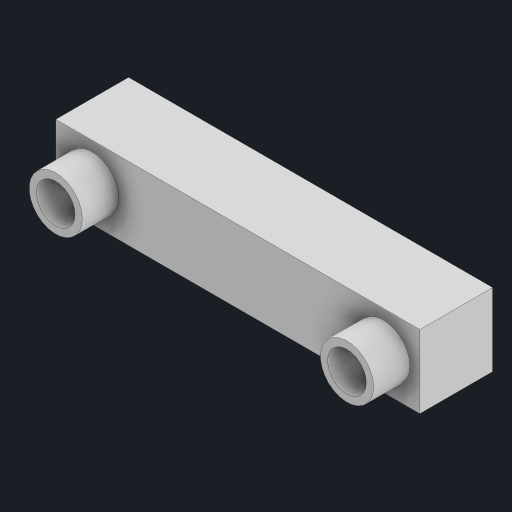
# Autodesk Inventor part: carriage_support
Saved by Autodesk Inventor 2024 (Build 280153000, 153)
## iProperties
Created: 2024-06-21
Part Number: carriage_support
Material: Generic
Document SubType Name: Modeling
Designer: mihir
Density: 1 g/cm^3
Appearance: Default
Author: mihir
Autodesk Inventor part; units mm, degrees
ref_plane "YZ Plane" through (0, 0, 0) normal (1, 0, 0) x (0, 1, 0)
ref_plane "XZ Plane" through (0, 0, 0) normal (0, 1, 0) x (-1, 0, 0)
ref_plane "XY Plane" through (0, 0, 0) normal (0, 0, 1) x (1, 0, 0)
sketch "Sketch1" plane through (0, 0, 0) normal (0, 1, 0) x (-1, 0, 0)
  line L0 (0, 0) -> (50, 0)
  line L1 (50, 0) -> (50, -10)
  line L2 (50, -10) -> (0, -10)
  line L3 (0, -10) -> (0, 0)
  dimension "d0" = 50
  dimension "d1" = 10
  constraints: 8 end point, 2 parallel, 1 horizontal, 1 perpendicular
  measures "d0" distance of L1.end L2.end
  measures "d1" distance of L2.end L0.start
extrude "Extrusion1" add sketch "Sketch1" along normal blind 10
sketch "Sketch2" plane through (-50, 0, 0) normal (0, 0, 1) x (1, 0, 0)
  circle A0 centre (5, 5) radius 2.65
  circle A1 centre (45, 5) radius 2.65
  line L0 (5, 5) -> (45, 5) construction
  line L1 (0, 10) -> (50, 10) construction
  line L2 (0, 0) -> (0, 10) construction
  circle A2 centre (5, 5) radius 3.65
  circle A3 centre (45, 5) radius 3.65
  point P0 (50, 0)
  dimension "d4" = 5
  dimension "d5" = 40
  dimension "d6" = 5
  dimension "d7" = 5.3
  dimension "d8" = 1
  constraints: 4 centre point, 2 coincident, 2 end point, 2 equal radius, 1 horizontal
  measures "d4" distance between parallel lines of L1 L0
  measures "d5" distance of L0.start L0.end
  measures "d6" distance from line of L2 L0.start
  measures "d7" diameter of A0
  measures "d8" radial gap between concentric circles of A2 A0
extrude "Extrusion2" add sketch "Sketch2" along normal blind 5
equation "\"d0\" = carriage_support_length"
equation "\"d1\" = carriage_support_width"
equation "\"d2\" = carriage_support_height"
equation "\"d4\" = 0.5 * carriage_support_height"
equation "\"d5\" = carriage_rod_dist"
equation "\"d6\" = 0.5 * carriage_support_length - 0.5 * carriage_rod_dist"
equation "\"d7\" = carriage_rod_diameter + rod_tolerance"
equation "\"carriage_rod_diameter\" = 5"
equation "\"rod_tolerance\" = 0.3"
equation "\"carriage_support_length\" = 50"
equation "\"carriage_support_width\" = 10"
equation "\"carriage_support_height\" = 10"
equation "\"carriage_rod_dist\" = 40"
body "Solid1"
